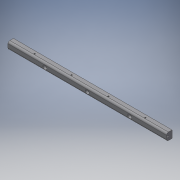
# Autodesk Inventor part: Wiper Springloaded 1_CPY
Saved by Autodesk Inventor 2019 (Build 230136000, 136)
## iProperties
Created: 2020-03-14
Part Number: Wiper Springloaded 1_CPY
Material: Generic
Document SubType Name: Modeling
Designer: Vijay
Density: 1 g/cm^3
Appearance: Default
Author: Vijay
Autodesk Inventor part; units mm, degrees
ref_plane "YZ Plane" through (0, 0, 0) normal (1, 0, 0) x (0, 1, 0)
ref_plane "XZ Plane" through (0, 0, 0) normal (0, 1, 0) x (-1, 0, 0)
ref_plane "XY Plane" through (0, 0, 0) normal (0, 0, 1) x (1, 0, 0)
sketch "Sketch1" plane through (0, 0, 0) normal (0, 0, 1) x (1, 0, 0)
  line L0 (-212.4247, -46.9955) -> (-212.4247, -61.9955) projected
  line L1 (-212.4247, -61.9955) -> (213.9753, -61.9955) projected
  line L2 (213.9753, -61.9955) -> (213.9753, -46.9955) projected
  line L3 (213.9753, -46.9955) -> (-212.4247, -46.9955) projected
  line L4 (213.9754, 278.5874) -> (243.9754, 278.5874) projected
  line L5 (243.9754, 278.5874) -> (243.9753, -71.9955) projected
  line L6 (243.9753, -71.9955) -> (-242.4247, -71.9955) projected
  line L7 (-242.4247, -71.9955) -> (-242.4246, 278.5875) projected
  line L8 (-242.4246, 278.5875) -> (-212.4246, 278.5875) projected
  line L9 (-212.4246, 278.5875) -> (-212.4247, -21.9955) projected
  line L10 (-212.4247, -21.9955) -> (213.9753, -21.9955) projected
  line L11 (213.9753, -21.9955) -> (213.9754, 278.5874) projected
  line L12 (-217.4247, -3.4496) -> (212.5753, -3.4496)
  line L13 (212.5753, -3.4496) -> (212.5753, 16.5504)
  line L14 (212.5753, 16.5504) -> (-217.4247, 16.5504)
  line L15 (-217.4247, 16.5504) -> (-217.4247, -3.4496)
  point P0 (0, 0)
  dimension "d1" = 20
  dimension "d11" = 430
  constraints: 8 end point, 2 parallel, 1 horizontal, 1 perpendicular
  measures "d1" distance between parallel lines of L14 L12
  measures "d11" distance of L13.end L14.end
extrude "Extrusion1" add sketch "Sketch1" along normal blind 15 contours L12 L15 L14 L9 | L9 L14 L13 L12
sketch "Sketch2" plane through (0, 0, 0) normal (0, 0, -1) x (-1, 0, 0)
  line L0 (217.4247, -3.4496) -> (-212.5753, -3.4496) construction
  line L1 (2.4247, -3.4496) -> (2.4247, 18.0985) construction
  line L2 (217.4247, 16.5504) -> (217.4247, -3.4496) construction
  line L3 (217.4247, 6.5504) -> (-212.5753, 6.5504) construction
  line L4 (-212.5753, -3.4496) -> (-212.5753, 16.5504) construction
  circle A0 centre (117.4247, 6.5504) radius 2.5
  circle A1 centre (-112.5753, 6.5504) radius 2.5
  circle A2 centre (2.4247, 6.5504) radius 2.5
  point P0 (0, 0)
  dimension "d4" = 5
  dimension "d5" = 100
  dimension "d6" = 5
  dimension "d7" = 100
  dimension "d8" = 5
  constraints: 4 end point, 4 midpoint, 3 centre point, 2 point on line, 1 vertical
  measures "d4" diameter of A0
  measures "d5" distance from line of L2 A0.centre
  measures "d6" diameter of A1
  measures "d7" distance from line of A1.centre L4
  measures "d8" diameter of A2
extrude "Extrusion2" cut sketch "Sketch2" against normal through all
sketch "Sketch3" plane through (0, 0, 15) normal (0, 0, 1) x (1, 0, 0)
  circle A0 centre (-117.4247, 6.5504) radius 2.5 projected
  circle A1 centre (-2.4247, 6.5504) radius 2.5 projected
  circle A2 centre (112.5753, 6.5504) radius 2.5 projected
  circle A3 centre (-117.4247, 6.5504) radius 5.5
  circle A4 centre (-2.4247, 6.5504) radius 5.5
  circle A5 centre (112.5753, 6.5504) radius 5.5
  point P0 (0, 0)
  dimension "d12" = 11
  dimension "d13" = 11
  dimension "d14" = 11
  constraints: 3 centre point, 3 coincident
  measures "d12" diameter of A3
  measures "d13" diameter of A4
  measures "d14" diameter of A5
extrude "Extrusion3" cut sketch "Sketch3" against normal blind 6 contours A0 | A1 | A2 | A3 | A4 | A5
sketch "Sketch4" plane through (212.5753, -3.4496, 0) normal (1, 0, 0) x (0, 0, -1)
  circle A0 centre (-11, 10) radius 2.1
  line L0 (-15, 0) -> (-15, 20) projected
  point P0 (0, 3.4496)
  dimension "d17" = 4.2
  dimension "d18" = 4
  constraints: 1 centre point
  measures "d17" diameter of A0
  measures "d18" distance from line of L0 A0.centre
extrude "Extrusion4" cut sketch "Sketch4" against normal blind 15
sketch "Sketch5" plane through (-217.4247, -3.4496, 0) normal (-1, 0, 0) x (0, 0, 1)
  circle A0 centre (11, 10) radius 2.1 projected
  circle A1 centre (11, 10) radius 2.1 projected
  point P0 (0, 3.4496)
extrude "Extrusion5" cut sketch "Sketch5" against normal blind 15
sketch "Sketch6" plane through (-217.4247, 16.5504, 0) normal (0, 1, 0) x (1, 0, 0)
  circle A0 centre (65, -7.4061) radius 1.75
  line L0 (430, 0) -> (0, 0) construction
  circle A1 centre (165, -7.4061) radius 1.75
  circle A2 centre (265, -7.4061) radius 1.75
  circle A3 centre (365, -7.4061) radius 1.75
  line L1 (0, 0) -> (0, -15) construction
  point P0 (217.4247, 0)
  dimension "d23" = 3.5
  dimension "d26" = 100
  dimension "d31" = 65
  constraints: 4 centre point, 1 horizontal, 6 other
  measures "d23" diameter of A0
  measures "d26" distance of A0.centre A1.centre
  measures "d31" distance from line of L1 A0.centre
extrude "Extrusion6" cut sketch "Sketch6" against normal through all
body "Solid1"
